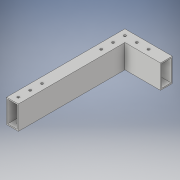
# Autodesk Inventor part: left arm
Saved by Autodesk Inventor 2018 (Build 220112000, 112)
## iProperties
Created: 2019-01-16
Part Number: left arm
Material: Generic
Document SubType Name: Modeling
Designer: s-4008082
Density: 1 g/cm^3
Appearance: Default
Author: s-4008082
Autodesk Inventor part; units mm, degrees
ref_plane "YZ Plane" through (0, 0, 0) normal (1, 0, 0) x (0, 1, 0)
ref_plane "XZ Plane" through (0, 0, 0) normal (0, 1, 0) x (-1, 0, 0)
ref_plane "XY Plane" through (0, 0, 0) normal (0, 0, 1) x (1, 0, 0)
sketch "Sketch15" plane through (0, 0, 0) normal (1, 0, 0) x (0, 1, 0)
  line L0 (0, 0) -> (50.8, 0)
  line L1 (50.8, 0) -> (50.8, 25.4)
  line L2 (50.8, 25.4) -> (0, 25.4)
  line L3 (0, 25.4) -> (0, 0)
  line L4 (48.26, 22.86) -> (2.54, 22.86)
  line L5 (2.54, 22.86) -> (2.54, 2.54)
  line L6 (2.54, 2.54) -> (48.26, 2.54)
  line L7 (48.26, 2.54) -> (48.26, 22.86)
  dimension "d46" = 25.4
  dimension "d47" = 50.8
  dimension "d48" = 2.54
  dimension "d49" = 2.54
  dimension "d50" = 2.54
  dimension "d51" = 2.54
  constraints: 16 end point, 4 parallel, 2 horizontal, 2 perpendicular
  measures "d46" distance of L0.end L1.end
  measures "d47" distance of L1.end L2.end
  measures "d48" distance between parallel lines of L1 L7
  measures "d49" distance between parallel lines of L2 L4
  measures "d50" distance between parallel lines of L3 L5
  measures "d51" distance between parallel lines of L0 L6
extrude "Extrusion12" add sketch "Sketch15" along normal blind 76.2
sketch "Sketch17" plane through (0, 0, 0) normal (0, 0, -1) x (-1, 0, 0)
  line L0 (0, 2.54) -> (-76.2, 2.54) projected
  line L1 (0, 48.26) -> (-76.2, 48.26) projected
  line L2 (-73.617, 2.54) -> (-3.1161, 2.54)
  line L3 (-3.1161, 2.54) -> (-3.1161, 48.26)
  line L4 (-3.1161, 48.26) -> (-73.617, 48.26)
  line L5 (-73.617, 48.26) -> (-73.617, 2.54)
  point P0 (0, 0)
  constraints: 8 end point, 2 parallel, 2 point on line, 1 horizontal, 1 perpendicular
extrude "Extrusion14" add sketch "Sketch17" along normal blind 2.54
sketch "Sketch20" plane through (0, 0, 0) normal (0, 0, -1) x (-1, 0, 0)
  line L0 (0, 0) -> (25.4, 0)
  line L1 (25.4, 0) -> (0, 0)
  line L2 (0, 0) -> (0, 50.8)
  line L3 (0, 50.8) -> (25.4, 50.8)
  line L4 (25.4, 50.8) -> (25.4, 0)
  line L5 (22.86, 48.26) -> (2.54, 48.26)
  line L6 (2.54, 48.26) -> (2.54, 2.54)
  line L7 (2.54, 2.54) -> (22.86, 2.54)
  line L8 (22.86, 2.54) -> (22.86, 48.26)
  line L9 (0, 0) -> (0, 50.8) projected
  dimension "d71" = 25.4
  dimension "d72" = 50.8
  dimension "d73" = 2.54
  dimension "d74" = 2.54
  dimension "d75" = 2.54
  dimension "d76" = 2.54
  dimension "d78" = 0
  constraints: 18 end point, 4 parallel, 2 horizontal, 2 perpendicular
  measures "d71" distance of L2.end L3.end
  measures "d72" distance of L1.end L2.end
  measures "d73" distance between parallel lines of L3 L5
  measures "d74" distance between parallel lines of L2 L6
  measures "d75" distance between parallel lines of L1 L7
  measures "d76" distance between parallel lines of L4 L8
  measures "d78" distance between parallel lines of L9 L2
extrude "Extrusion16" add sketch "Sketch20" against normal blind 254
sketch "Sketch21" plane through (76.2, 0, 0) normal (0, -1, 0) x (1, 0, 0)
  circle A0 centre (-38.1, 12.7) radius 2.5797
  circle A1 centre (-63.5, 12.7) radius 2.5797
  circle A2 centre (-88.9, 12.7) radius 2.5797
  circle A3 centre (-88.9, 38.1) radius 2.5797
  circle A4 centre (-88.9, 63.5) radius 2.5797
  line L0 (-76.2, 25.4) -> (0, 25.4) projected
  line L1 (-101.6, 0) -> (-101.6, 254) projected
  line L2 (-76.2, 25.4) -> (-76.2, 254) projected
  point P0 (-76.2, 0)
  dimension "d81" = 12.7
  dimension "d82" = 12.7
  dimension "d83" = 12.7
  dimension "d84" = 25.4
  dimension "d85" = 12.7
  dimension "d86" = 5.1594
  dimension "d87" = 5.1594
  dimension "d88" = 5.1594
  dimension "d89" = 25.4
  dimension "d90" = 25.4
  dimension "d91" = 25.4
  dimension "d92" = 5.1594
  dimension "d93" = 5.1594
  dimension "d94" = 12.7
  dimension "d95" = 12.7
  constraints: 5 centre point
  measures "d81" distance from line of L0 A0.centre
  measures "d82" distance from line of L0 A2.centre
  measures "d83" distance from line of L1 A2.centre
  measures "d84" distance of A2.centre A1.centre
  measures "d85" distance from line of L0 A1.centre
  measures "d86" diameter of A0
  measures "d87" diameter of A1
  measures "d88" diameter of A2
  measures "d89" distance of A1.centre A0.centre
  measures "d90" distance of A2.centre A3.centre
  measures "d91" distance of A3.centre A4.centre
  measures "d92" diameter of A4
  measures "d93" diameter of A3
  measures "d94" distance from line of L2 A3.centre
  measures "d95" distance from line of L2 A4.centre
extrude "Extrusion17" cut sketch "Sketch21" against normal blind 76.2
sketch "Sketch22" plane through (76.2, 50.8, 25.4) normal (0, 1, 0) x (1, 0, 0)
  circle A0 centre (-88.9, -215.9) radius 2.5797
  circle A1 centre (-88.9, -190.5) radius 2.5797
  circle A2 centre (-88.9, -165.1) radius 2.5797
  line L0 (-76.2, 0) -> (-76.2, -228.6) projected
  line L1 (-76.2, -228.6) -> (-101.6, -228.6) projected
  point P0 (-76.2, 25.4)
  dimension "d98" = 25.4
  dimension "d99" = 25.4
  dimension "d100" = 12.7
  dimension "d101" = 12.7
  dimension "d102" = 12.7
  dimension "d103" = 5.1594
  dimension "d104" = 5.1594
  dimension "d105" = 5.1594
  dimension "d108" = 12.7
  constraints: 3 centre point
  measures "d98" distance of A1.centre A0.centre
  measures "d99" distance of A1.centre A2.centre
  measures "d100" distance from line of L0 A0.centre
  measures "d101" distance from line of L0 A1.centre
  measures "d102" distance from line of L0 A2.centre
  measures "d103" diameter of A0
  measures "d104" diameter of A1
  measures "d105" diameter of A2
  measures "d108" distance from line of L1 A0.centre
extrude "Extrusion18" cut sketch "Sketch22" against normal blind 76.2
equation "\"d49\" = d48"
equation "\"d50\" = d48"
equation "\"d51\" = d48"
equation "\"d73\" = d77"
equation "\"d74\" = d77"
equation "\"d75\" = d77"
equation "\"d76\" = d77"
equation "\"d87\" = d86"
equation "\"d88\" = d86"
equation "\"d92\" = d86"
equation "\"d93\" = d86"
equation "\"d101\" = d100"
equation "\"d102\" = d100"
equation "\"d104\" = d103"
equation "\"d105\" = d103"
equation "\"d77\" = 2.54"
body "Solid2"
